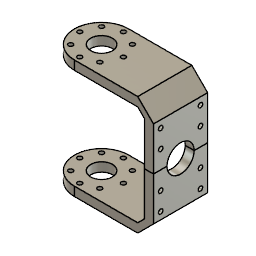
_Rotating Bracket.902a2a08-6bf0-4443-ad28-58b1b6e1e9f1 (Autodesk Fusion 360 design; units mm, degrees)
Autodesk Fusion 360 part; units mm, degrees
sketch "Sketch1" plane through (0, 0, 0) normal (0, 1, 0) x (1, 0, 0)
  circle A0 centre (0, 0) radius 6
  line L0 (0, 15) -> (35, 15)
  line L1 (35, 15) -> (35, -15)
  line L2 (35, -15) -> (0, -15)
  arc A1 (0, 15) -> (0, -15) centre (0, 0) ccw
  circle A2 centre (-12.081, 0) radius 1.25
  circle A3 centre (0, 12.081) radius 1.25
  circle A4 centre (0, -12.081) radius 1.25
  circle A5 centre (12.081, 0) radius 1.25
  circle A6 centre (8.4947, 8.5902) radius 1.25
  circle A7 centre (-8.5426, 8.5426) radius 1.25
  circle A8 centre (-8.4947, -8.5902) radius 1.25
  circle A9 centre (8, -9) radius 1.25
  dimension "d2" = 30
  dimension "d3" = 12
  dimension "d4" = 2.5
  dimension "d6" = 35
  dimension "d7" = 12.081
  dimension "d8" = 2.5
  dimension "d9" = 2.5
  dimension "d10" = 2.5
  dimension "d11" = 12.081
  dimension "d12" = 12.081
  dimension "d13" = 12.081
  dimension "d14" = 2.5
  dimension "d15" = 2.5
  dimension "d16" = 12.081
  dimension "d17" = 12.081
  dimension "d18" = 2.5
  dimension "d19" = 2.5
  dimension "d20" = 12.081
  dimension "d21" = 9.184
  constraint coincident A0.centre A1.centre
  constraint tangent L0 A1
  constraint horizontal L0
  constraint perpendicular L0 L1
  constraint tangent L2 A1
  constraint perpendicular L1 L2
  constraint horizontal A0.centre A2.centre
  constraint vertical L2.end A4.centre
  constraint vertical L2.end A3.centre
  constraint horizontal A2.centre A5.centre
  measures "d2" diameter of A1
  measures "d3" diameter of A0
  measures "d4" diameter of A2
  measures "d6" distance of A0.centre L1
  measures "d7" distance of A0.centre A2.centre
  measures "d8" diameter of A3
  measures "d9" diameter of A4
  measures "d10" diameter of A5
  measures "d11" distance of A0.centre A3.centre
  measures "d12" distance of A0.centre A4.centre
  measures "d13" distance of A0.centre A5.centre
  measures "d14" diameter of A6
  measures "d15" diameter of A7
  measures "d16" distance of A0.centre A7.centre
  measures "d17" distance of A0.centre A6.centre
  measures "d18" diameter of A8
  measures "d19" diameter of A9
  measures "d20" distance of A0.centre A8.centre
  measures "d21" distance of A3.centre A6.centre
extrude "Extrude1" add sketch "Sketch1" along normal blind 5 makes body 1
sketch "Sketch2" plane through (0, 0, 15) normal (0, 0, 1) x (1, 0, 0)
  line L0 (0, 0) -> (35, 0)
  line L1 (35, 0) -> (35, 5)
  line L2 (35, 5) -> (0, 5)
  line L3 (0, 5) -> (0, 0)
  line L4 (35, 5) -> (43.75, -3.75)
  line L5 (35, 5) -> (49.1421, 5) construction
  line L6 (35, 0) -> (43.75, -8.75)
  line L7 (35, 0) -> (47.3744, 0) construction
  line L8 (43.75, -3.75) -> (43.75, -8.75)
  dimension "d26" = 45
  dimension "d27" = 8.75
  dimension "d28" = 45
  constraint horizontal L5
  constraint coincident L1.end L2.start
  constraint horizontal L7
  constraint coincident L0.end L1.start
  constraint equal L6 L7
  constraint equal L4 L6
  measures "d26" angle of L4 L5
  measures "d27" distance of L2 L4.end
  measures "d28" angle of L6 L7
extrude "Extrude2" add sketch "Sketch2" against normal blind 30 contours L1 L4 L6 L8 bodies 1
sketch "Sketch3" plane through (0, 0, 15) normal (0, 0, 1) x (1, 0, 0)
  line L0 (0, 0) -> (35, 0)
  line L1 (35, 0) -> (43.75, -8.75)
  line L2 (43.75, -8.75) -> (43.75, -3.75)
  line L3 (43.75, -3.75) -> (35, 5)
  line L4 (35, 5) -> (0, 5)
  line L5 (0, 5) -> (0, 0)
  line L6 (43.75, -3.75) -> (38.75, -3.75)
  line L7 (38.75, -3.75) -> (38.75, -27.75)
  line L8 (38.75, -27.75) -> (43.75, -27.75)
  line L9 (43.75, -27.75) -> (43.75, -3.75)
  dimension "d31" = 5
  dimension "d32" = 24
  constraint horizontal L6
  constraint vertical L7
  constraint horizontal L8
  constraint vertical L9
  constraint coincident L2.end L3.start
  measures "d31" distance of L2.end L6.end
  measures "d32" distance of L2.end L8.end
extrude "Extrude3" add sketch "Sketch3" against normal blind 30 contours L1 L7 L8 L9 bodies 1
sketch "Sketch5" plane through (43.75, 0, 0) normal (1, 0, 0) x (0, 0, -1)
  line L0 (-15, -3.75) -> (-15, -27.75)
  line L1 (-15, -27.75) -> (15, -27.75)
  line L2 (15, -27.75) -> (15, -3.75)
  line L3 (15, -3.75) -> (-15, -3.75)
  circle A0 centre (-11, -7.75) radius 1.25
  circle A1 centre (11, -7.75) radius 1.25
  circle A2 centre (-11, -17.75) radius 1.25
  circle A3 centre (11, -17.75) radius 1.25
  circle A4 centre (0, -27.75) radius 7.5
  dimension "d53" = 2.5
  dimension "d54" = 2.5
  dimension "d55" = 2.5
  dimension "d56" = 2.5
  dimension "d57" = 15
  dimension "d58" = 4
  dimension "d59" = 4
  dimension "d60" = 4
  dimension "d61" = 10
  dimension "d62" = 4
  dimension "d63" = 4
  dimension "d64" = 10
  dimension "d65" = 4
  constraint midpoint L1 A4.centre
  measures "d53" diameter of A0
  measures "d54" diameter of A1
  measures "d55" diameter of A2
  measures "d56" diameter of A3
  measures "d57" diameter of A4
  measures "d58" distance of L3 A0.centre
  measures "d59" distance of L0 A0.centre
  measures "d60" distance of L0 A2.centre
  measures "d61" distance of A0.centre A2.centre
  measures "d62" distance of L3 A1.centre
  measures "d63" distance of L2 A1.centre
  measures "d64" vertical distance of A1.centre A3.centre
  measures "d65" distance of L2 A3.centre
extrude "Extrude5" cut sketch "Sketch5" against normal blind 5 contours L1 A4 | A0 | A1 | A2 | A3 picked at (-0.5563, -25.3127) bodies 1
ref_plane "WorkPlane2" through (38.75, -27.75, 15) normal (0, -1, 0) x (1, 0, 0)
mirror "Mirror2" about plane through (38.75, -27.75, 15) normal (0, -1, 0) of bodies 1 makes body 2
